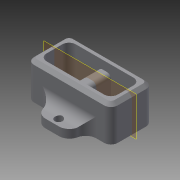
# Autodesk Inventor part: Single Mount
Saved by Autodesk Inventor 2015 (Build 190159000, 159)
## iProperties
Created: 2015-04-19
Part Number: Single Mount
Material: Generic
Document SubType Name: Modeling
Designer: Kyle
Density: 1 g/cm^3
Appearance: Default
Author: Kyle
Autodesk Inventor part; units mm, degrees
ref_plane "YZ Plane" through (0, 0, 0) normal (1, 0, 0) x (0, 1, 0)
ref_plane "XZ Plane" through (0, 0, 0) normal (0, 1, 0) x (-1, 0, 0)
ref_plane "XY Plane" through (0, 0, 0) normal (0, 0, 1) x (1, 0, 0)
sketch "Sketch1" plane through (0, 0, 0) normal (0, 1, 0) x (-1, 0, 0)
  line L0 (-12.7, 6.35) -> (12.7, 6.35)
  line L1 (12.7, 6.35) -> (12.7, -6.35)
  line L2 (12.7, -6.35) -> (-12.7, -6.35)
  line L3 (-12.7, -6.35) -> (-12.7, 6.35)
  line L4 (-12.7, 6.35) -> (12.7, -6.35) construction
  line L5 (12.7, 6.35) -> (-12.7, -6.35) construction
  point P0 (0, 0)
  point P1 (0, 0)
  dimension "d0" = 12.7
  dimension "d1" = 25.4
  constraints: 12 end point, 4 midpoint, 2 parallel, 1 horizontal, 1 perpendicular
  measures "d0" distance of L0.end L1.end
  measures "d1" distance of L1.end L2.end
extrude "Extrusion1" add sketch "Sketch1" along normal blind 9.525 and the other way blind 1.27
sketch "Sketch2" plane through (0, 9.525, 0) normal (0, 1, 0) x (1, 0, 0)
  line L0 (-10.795, -4.445) -> (10.795, -4.445)
  line L1 (10.795, -4.445) -> (10.795, 4.445)
  line L2 (10.795, 4.445) -> (-10.795, 4.445)
  line L3 (-10.795, 4.445) -> (-10.795, -4.445)
  line L4 (-10.795, -4.445) -> (10.795, 4.445) construction
  line L5 (10.795, -4.445) -> (-10.795, 4.445) construction
  point P0 (0, 0)
  dimension "d6" = 21.59
  dimension "d7" = 8.89
  constraints: 12 end point, 2 midpoint, 2 parallel, 1 horizontal, 1 perpendicular
  measures "d6" distance of L1.end L2.end
  measures "d7" distance of L0.end L1.end
extrude "Extrusion2" cut sketch "Sketch2" against normal blind 2.54
sketch "Sketch3" plane through (0, 6.985, 0) normal (0, 1, 0) x (1, 0, 0)
  line L0 (10.795, -4.445) -> (-10.795, -4.445) projected
  line L1 (-10.795, 4.445) -> (-1.905, 4.445)
  line L2 (-1.905, 4.445) -> (-1.905, -4.445)
  line L3 (-1.905, -4.445) -> (-10.795, -4.445)
  line L4 (-10.795, -4.445) -> (-10.795, 4.445)
  line L5 (10.795, 4.445) -> (1.905, 4.445)
  line L6 (1.905, 4.445) -> (1.905, -4.445)
  line L7 (1.905, -4.445) -> (10.795, -4.445)
  line L8 (10.795, -4.445) -> (10.795, 4.445)
  point P0 (0, 0)
  dimension "d10" = 8.89
  dimension "d11" = 8.89
  dimension "d12" = 8.89
  dimension "d13" = 8.89
  constraints: 16 end point, 4 parallel, 2 horizontal, 2 perpendicular, 2 point on line
  measures "d10" distance of L1.start L1.end
  measures "d11" distance of L3.end L1.start
  measures "d12" distance of L5.start L5.end
  measures "d13" distance of L7.end L5.start
extrude "Extrusion3" cut sketch "Sketch3" against normal blind 6.35
sketch "Sketch4" plane through (0, 0.635, 0) normal (0, 1, 0) x (1, 0, 0)
  line L0 (0, 0) -> (-6.35, 0) construction
  line L1 (-6.35, 0) -> (-6.35, 2.54) construction
  line L2 (-6.35, 0) -> (-6.35, -2.54) construction
  line L3 (0, 0) -> (6.35, 0) construction
  line L4 (6.35, 0) -> (6.35, 2.54) construction
  line L5 (6.35, 0) -> (6.35, -2.54) construction
  circle A0 centre (-6.35, 2.54) radius 1.27
  circle A1 centre (-6.35, -2.54) radius 1.27
  circle A2 centre (6.35, -2.54) radius 1.27
  circle A3 centre (6.35, 2.54) radius 1.27
  dimension "d16" = 2.54
  dimension "d17" = 6.35
  dimension "d18" = 2.54
  constraints: 12 end point, 4 centre point, 4 coincident, 4 equal length, 3 equal radius, 2 horizontal, 2 perpendicular, 2 vertical
  measures "d16" distance of L0.end L1.end
  measures "d17" distance of L0.start L0.end
  measures "d18" diameter of A0
extrude "Extrusion4" cut sketch "Sketch4" along normal mid plane 6.35
sketch "Sketch5" plane through (0, -1.27, 0) normal (0, -1, 0) x (1, 0, 0)
  line L0 (-12.7, 6.35) -> (12.7, 6.35) projected
  line L1 (-5.08, 6.35) -> (5.08, 6.35)
  line L2 (5.08, 6.35) -> (5.08, 11.43)
  line L3 (5.08, 11.43) -> (-5.08, 11.43)
  line L4 (-5.08, 11.43) -> (-5.08, 6.35)
  line L5 (0, 0) -> (0, 9.27) construction
  line L6 (0, 0) -> (-15.0556, 0) construction
  dimension "d21" = 10.16
  dimension "d22" = 5.08
  constraints: 12 end point, 2 horizontal, 2 parallel, 1 perpendicular, 1 point on line, 1 vertical, 1 other
  measures "d21" distance of L2.end L3.end
  measures "d22" distance of L3.end L1.start
extrude "Extrusion5" add sketch "Sketch5" against normal blind 2.54
ref_plane "Work Plane1" through (-10.795, 9.525, 0) normal (0, 0, 1) x (1, 0, 0)
mirror "Mirror1" about plane through (-10.795, 9.525, 0) normal (0, 0, 1) of "Extrusion5"
fillet "Fillet1" radius 3.175 5 edges at (0, 1.27, 6.35) (-5.08, 0, 11.43) (5.08, 0, 11.43) (5.08, 0, 6.35) (-5.08, 0, 6.35)
fillet "Fillet2" radius 3.175 5 edges at (0, 1.27, -6.35) (5.08, 0, -11.43) (-5.08, 0, -11.43) (-5.08, 0, -6.35) (5.08, 0, -6.35)
fillet "Fillet3" radius 2.032 8 edges at (-10.795, 5.08, 4.445) (-10.795, 5.08, -4.445) (10.795, 5.08, -4.445) (10.795, 5.08, 4.445) (12.7, 4.1275, -6.35) (-12.7, 4.1275, -6.35) (-12.7, 4.1275, 6.35) (12.7, 4.1275, 6.35)
fillet "Fillet4" radius 1.27 1 edges at (1.905, 6.985, 0)
fillet "Fillet5" radius 1.27 1 edges at (-1.905, 6.985, 0)
sketch "Sketch6" plane through (0, 0.635, 0) normal (0, 1, 0) x (1, 0, 0)
  line L0 (-4.9432, -9.525) -> (4.9432, -9.525) projected
  circle A0 centre (0, -9.525) radius 1.1645
  circle A1 centre (0, -9.525) radius 1.1645
  line L1 (0, 0) -> (16.6664, 0) construction
  circle A2 centre (0, 9.525) radius 1.1645
  constraints: 3 centre point, 2 end point, 1 coincident, 1 horizontal, 1 midpoint, 1 symmetric about line, 1 other
extrude "Extrusion6" cut sketch "Sketch6" along normal mid plane 6.35
chamfer "Chamfer1" distance 0.9525 angle 45 8 edges at (0, 9.525, -6.35) (-12.1048, 9.525, -5.7548) (-12.7, 9.525, 0) (-12.1048, 9.525, 5.7548) (0, 9.525, 6.35) (12.1048, 9.525, 5.7548) (12.7, 9.525, 0) (12.1048, 9.525, -5.7548)
body "Solid1"
